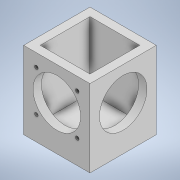
# Autodesk Inventor part: immersion_chamber_bath
Saved by Autodesk Inventor 2021 (Build 250183000, 183)
## iProperties
Created: 2021-06-16
Part Number: immersion_chamber_bath
Material: Generic
Document SubType Name: Modeling
Designer: MicroscopyInnovation
Density: 1 g/cm^3
Appearance: Default
Author: MicroscopyInnovation
Autodesk Inventor part; units mm, degrees
ref_plane "YZ Plane" through (0, 0, 0) normal (1, 0, 0) x (0, 1, 0)
ref_plane "XZ Plane" through (0, 0, 0) normal (0, 1, 0) x (-1, 0, 0)
ref_plane "XY Plane" through (0, 0, 0) normal (0, 0, 1) x (1, 0, 0)
sketch "Sketch1" plane through (0, 0, 0) normal (0, 1, 0) x (-1, 0, 0)
  line L0 (-30, 30) -> (30, 30)
  line L1 (30, 30) -> (30, -30)
  line L2 (30, -30) -> (-30, -30)
  line L3 (-30, -30) -> (-30, 30)
  line L4 (-30, 30) -> (30, -30) construction
  line L5 (30, 30) -> (-30, -30) construction
  point P0 (0, 0)
  dimension "d0" = 60
  dimension "d1" = 60
  constraints: 12 end point, 2 midpoint, 2 parallel, 1 horizontal, 1 perpendicular
  measures "d0" distance of L1.end L2.end
  measures "d1" distance of L0.end L1.end
extrude "Extrusion1" add sketch "Sketch1" along normal blind 70
sketch "Sketch2" plane through (0, 70, 0) normal (0, 1, 0) x (1, 0, 0)
  line L0 (22.5, 22.5) -> (-22.5, 22.5)
  line L1 (-22.5, 22.5) -> (-22.5, -22.5)
  line L2 (-22.5, -22.5) -> (22.5, -22.5)
  line L3 (22.5, -22.5) -> (22.5, 22.5)
  line L4 (22.5, 22.5) -> (-22.5, -22.5) construction
  line L5 (-22.5, 22.5) -> (22.5, -22.5) construction
  point P0 (0, 0)
  dimension "d4" = 45
  dimension "d5" = 45
  constraints: 12 end point, 2 midpoint, 2 parallel, 1 horizontal, 1 perpendicular
  measures "d4" distance of L2.end L1.end
  measures "d5" distance of L1.end L0.end
extrude "Extrusion2" cut sketch "Sketch2" against normal blind 60
sketch "Sketch3" plane through (-30, 0, 30) normal (0, 0, 1) x (1, 0, 0)
  circle A0 centre (30, 40) radius 21.5
  point P0 (30, 0)
  dimension "d8" = 43
  constraints: 1 centre point
  measures "d8" diameter of A0
extrude "Extrusion3" cut sketch "Sketch3" against normal blind 15
sketch "Sketch4" plane through (30, 0, 30) normal (1, 0, 0) x (0, 0, -1)
  circle A0 centre (30, 40) radius 21.5
  point P0 (30, 0)
  dimension "d11" = 43
  constraints: 1 centre point
  measures "d11" diameter of A0
extrude "Extrusion4" cut sketch "Sketch4" against normal blind 15
sketch "Sketch5" plane through (0, 0, 0) normal (0, -1, 0) x (1, 0, 0)
  point P0 (0, 0)
  point P1 (0, 0)
  constraints: 1 coincident
hole "Hole1" at (0, 0, 0) direction (0, 1, 0) diameter 3.302 depth 8 thread size "8-32 UNC" class "2B" standard "ANSI Unified Screw Threads"
sketch "Sketch7" plane through (-30, 0, 30) normal (0, 0, 1) x (1, 0, 0)
  line L0 (11.5, 21.5) -> (48.5, 21.5)
  line L1 (48.5, 21.5) -> (48.5, 58.5)
  line L2 (48.5, 58.5) -> (11.5, 58.5)
  line L3 (11.5, 58.5) -> (11.5, 21.5)
  line L4 (11.5, 21.5) -> (48.5, 58.5) construction
  line L5 (48.5, 21.5) -> (11.5, 58.5) construction
  point P0 (30, 0)
  point P1 (30, 40)
  dimension "d21" = 37
  dimension "d22" = 37
  constraints: 12 end point, 2 midpoint, 2 parallel, 1 horizontal, 1 perpendicular
  measures "d21" distance of L2.end L1.end
  measures "d22" distance of L1.end L0.end
hole "Hole2" at (-18.5, 58.5, 30) at (18.5, 58.5, 30) at (18.5, 21.5, 30) at (-18.5, 21.5, 30) direction (0, 0, -1) diameter 3.302 depth 6 thread size "8-32 UNC" class "2B" standard "ANSI Unified Screw Threads"
body "Solid1"
